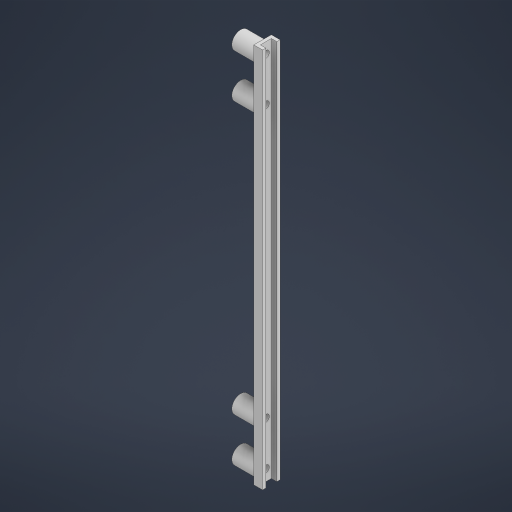
# Autodesk Inventor part: hs_intake_front_brace
Saved by Autodesk Inventor 2024 (Build 280153000, 153)
## iProperties
Created: 2023-10-10
Part Number: hs_intake_front_brace
Material: Generic
Document SubType Name: Modeling
Designer: Averey Ku
Density: 1 g/cm^3
Appearance: Default
Author: Averey Ku
Autodesk Inventor part; units mm, degrees
ref_plane "YZ Plane" through (0, 0, 0) normal (1, 0, 0) x (0, 1, 0)
ref_plane "XZ Plane" through (0, 0, 0) normal (0, 1, 0) x (-1, 0, 0)
ref_plane "XY Plane" through (0, 0, 0) normal (0, 0, 1) x (1, 0, 0)
sketch "Sketch1" plane through (0, 0, 0) normal (0, 1, 0) x (-1, 0, 0)
  line L0 (0, 3.1877) -> (3.1877, 3.1877)
  line L1 (3.1877, 3.1877) -> (3.1877, -3.1877)
  line L2 (3.1877, -3.1877) -> (0, -3.1877)
  line L3 (0, 5.08) -> (5.08, 5.08)
  line L4 (5.08, 5.08) -> (5.08, -5.08)
  line L5 (5.08, -5.08) -> (0, -5.08)
  line L6 (0, -5.08) -> (0, -3.1877)
  line L7 (0, 3.1877) -> (0, 5.08)
  point P0 (0, 0)
  dimension "d0" = 3.1877
  dimension "d1" = 6.3754
  dimension "d2" = 5.08
  dimension "d3" = 10.16
  constraints: 16 end point, 4 parallel, 2 horizontal, 2 perpendicular
  measures "d0" distance of L1.end L2.end
  measures "d1" distance of L0.end L1.end
  measures "d2" distance of L4.end L5.end
  measures "d3" distance of L3.end L4.end
extrude "Extrusion1" add sketch "Sketch1" along normal blind 220.5736
sketch "Sketch2" plane through (-5.08, 0, -5.08) normal (-1, 0, 0) x (0, 0, 1)
  circle A0 centre (5.08, 6.35) radius 1.9844
  circle A1 centre (5.08, 214.2236) radius 1.9844
  circle A2 centre (5.08, 31.75) radius 1.9844
  circle A3 centre (5.08, 188.8236) radius 1.9844
  point P0 (5.08, 0)
  dimension "d6" = 3.9688
  dimension "d7" = 3.9688
  dimension "d12" = 3.9688
  dimension "d13" = 3.9688
  constraints: 4 centre point
  measures "d6" diameter of A0
  measures "d7" diameter of A1
  measures "d12" diameter of A2
  measures "d13" diameter of A3
sketch "Sketch3" plane through (-5.08, 0, -5.08) normal (-1, 0, 0) x (0, 0, 1)
  point P0 (5.08, 0)
extrude "Extrusion4" cut sketch "Sketch2" against normal blind 12.7
sketch "Sketch5" plane through (-5.08, 6.35, 0) normal (-1, 0, 0) x (0, 0, 1)
  circle A0 centre (0, 0) radius 1.9844 projected
  circle A1 centre (0, 25.4) radius 1.9844 projected
  circle A2 centre (0, 182.4736) radius 1.9844 projected
  circle A3 centre (0, 207.8736) radius 1.9844 projected
  circle A4 centre (0, 0) radius 5.08
  line L0 (-5.08, -6.35) -> (-5.08, 214.2236) projected
  circle A5 centre (0, 25.4) radius 5.08
  circle A6 centre (0, 207.8736) radius 5.08
  circle A7 centre (0, 182.4736) radius 5.08
  point P0 (0, -6.35)
  constraints: 4 centre point, 4 coincident, 1 tangent
extrude "Extrusion5" add sketch "Sketch5" along normal blind 12.7
body "Solid1"
